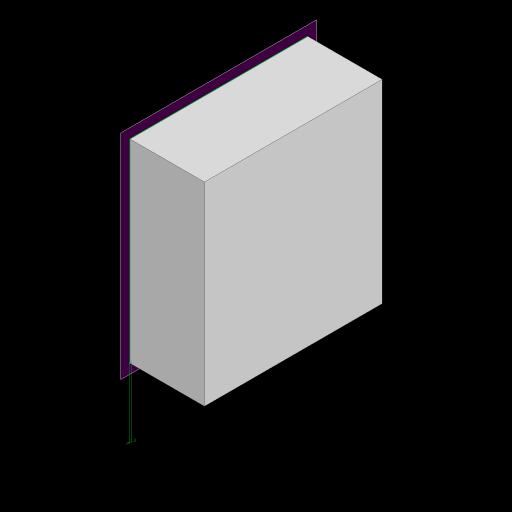
# Autodesk Inventor part: wooferBox
Saved by Autodesk Inventor 2023 (Build 270158000, 158)
## iProperties
Created: 2022-07-12
Part Number: wooferBox
Material: Generic
Document SubType Name: Modeling
Designer: Fuzzyfish
Density: 1 g/cm^3
Appearance: Default
Author: Fuzzyfish
Autodesk Inventor part; units mm, degrees
ref_plane "YZ Plane" through (0, 0, 0) normal (1, 0, 0) x (0, 1, 0)
ref_plane "XZ Plane" through (0, 0, 0) normal (0, 1, 0) x (-1, 0, 0)
ref_plane "XY Plane" through (0, 0, 0) normal (0, 0, 1) x (1, 0, 0)
sketch "Sketch1" plane through (0, 0, 0) normal (0, 1, 0) x (-1, 0, 0)
  line L0 (0, 0) -> (100, 0)
  line L1 (100, 0) -> (100, -119)
  line L2 (100, -119) -> (0, -119)
  line L3 (0, -119) -> (0, 0)
  dimension "d0" = 119
  dimension "d1" = 100
  constraints: 8 end point, 2 parallel, 1 horizontal, 1 perpendicular
  measures "d0" distance between parallel lines of L2 L0
  measures "d1" distance of L1.end L2.end
extrude "Extrusion1" add sketch "Sketch1" along normal blind 130
sketch "Sketch2" plane through (0, 0, -119) normal (0, 0, -1) x (-1, 0, 0)
  circle A0 centre (50, 65) radius 45
  line L0 (100, 0) -> (100, 130) projected
  line L1 (0, 0) -> (0, 130) projected
  line L2 (0, 0) -> (100, 0) projected
  line L3 (0, 130) -> (100, 130) projected
  circle A1 centre (50, 65) radius 36.5
  circle A2 centre (28.0236, 99.1226) radius 1.9
  line L4 (25.6342, 102.8326) -> (74.3658, 27.1674) construction
  line L5 (12.1674, 40.6342) -> (87.8326, 89.3658) construction
  dimension "d6" = 90
  dimension "d7" = 100
  dimension "d8" = 50
  dimension "d9" = 65
  dimension "d10" = 130
  dimension "d11" = 73
  dimension "d12" = 3.8
  constraints: 4 end point, 4 point on circle, 3 centre point, 2 line through centre, 1 coincident, 1 perpendicular, 1 point on line
  measures "d6" diameter of A0
  measures "d7" distance between parallel lines of L0 L1
  measures "d8" distance from line of L1 A0.centre
  measures "d9" distance from line of L2 A0.centre
  measures "d10" distance between parallel lines of L2 L3
  measures "d11" diameter of A1
  measures "d12" diameter of A2
extrude "Extrusion2" cut sketch "Sketch2" against normal blind 8 contours A0 | A1 | A2
extrude "Extrusion3" cut sketch "Sketch2" against normal blind 18 contours A1
ref_plane "Work Plane1" through (-95, 0, -119) normal (-1, 0, 0) x (0, 0, 1)
sketch "Sketch3" plane through (-95, 0, -119) normal (-1, 0, 0) x (0, 0, 1)
  line L0 (18, 28.5) -> (18, 101.5) projected
  line L1 (119, 130) -> (119, 0) projected
  line L2 (119, 0) -> (0, 0) projected
  line L3 (0, 0) -> (0, 65) projected
  line L4 (8, 65) -> (0, 65) projected
  line L5 (0, 130) -> (119, 130) projected
  line L6 (0, 65) -> (0, 130) projected
  line L7 (114, 125) -> (18, 125)
  line L8 (18, 125) -> (18, 5)
  line L9 (18, 5) -> (114, 5)
  line L10 (114, 5) -> (114, 125)
  dimension "d16" = 5
  dimension "d17" = 5
  dimension "d18" = 5
  constraints: 8 end point, 2 parallel, 1 collinear, 1 horizontal, 1 perpendicular
  measures "d16" distance between parallel lines of L2 L9
  measures "d17" distance between parallel lines of L1 L10
  measures "d18" distance between parallel lines of L5 L7
extrude "Extrusion4" cut sketch "Sketch3" against normal blind 90 contours L0 L8 L7 L10 L9
fillet "Fillet1" radius 5 12 edges at (-50, 5, -5) (-5, 5, -53) (-5, 65, -5) (-5, 125, -53) (-50, 125, -5) (-95, 125, -53) (-95, 65, -5) (-95, 5, -53) (-50, 5, -101) (-50, 125, -101) (-95, 65, -101) (-5, 65, -101)
sketch "Sketch8" plane through (-100, 0, -119) normal (-1, 0, 0) x (0, 0, 1)
  point P0 (119, 0)
sketch "Sketch10" plane through (-100, 0, -119) normal (-1, 0, 0) x (0, 0, 1)
  line L0 (0, 0) -> (119, 0) projected
  line L1 (119, 0) -> (119, 130) projected
  line L2 (0, 130) -> (119, 130) projected
  line L3 (0, 0) -> (0, 130) projected
extrude "Extrusion10" add sketch "Sketch10" along normal blind 5
sketch "Sketch12" plane through (0, 130, 0) normal (0, 1, 0) x (1, 0, 0)
  line L0 (0, 119) -> (-105, 119) projected
  line L1 (-105, 0) -> (-105, 119) projected
  line L2 (0, 0) -> (-105, 0) projected
  line L3 (0, 0) -> (0, 119) projected
  line L4 (-105, 0) -> (-100, 0)
  line L5 (-100, 0) -> (-100, 119)
  line L6 (-100, 119) -> (-105, 119)
  line L7 (-105, 119) -> (-105, 0)
  line L8 (-100, 20) -> (-105, 25)
  line L9 (-105, 40) -> (-100, 45)
  line L10 (-105, 94) -> (-100, 99)
  line L11 (-100, 74) -> (-105, 79)
  dimension "d82" = 119
  dimension "d86" = 5
  dimension "d87" = 45
  dimension "d88" = 45
  dimension "d90" = 45
  dimension "d91" = 45
  dimension "d92" = 20
  dimension "d93" = 25
  dimension "d94" = 20
  dimension "d95" = 25
  constraints: 16 end point, 9 point on line, 2 parallel, 1 horizontal, 1 perpendicular
  measures "d82" distance of L0.end L1.start
  measures "d86" distance between parallel lines of L1 L5
  measures "d87" angle of L5 L8
  measures "d88" angle of L5 L9
  measures "d90" angle of L5 L11
  measures "d91" angle of L5 L10
  measures "d92" distance of L4.end L8.start
  measures "d93" distance of L9.end L8.start
  measures "d94" distance of L5.end L10.end
  measures "d95" distance of L11.start L10.end
extrude "Extrusion11" cut sketch "Sketch12" against normal blind 127 contours L5 L11 L1 L10 | L8 L1 L9 L5
fillet "Fillet2" radius 1 8 edges at (-105, 66.5, -25) (-100, 66.5, -20) (-105, 66.5, -40) (-100, 66.5, -45) (-105, 66.5, -79) (-100, 66.5, -74) (-105, 66.5, -94) (-100, 66.5, -99)
sketch "Sketch13" plane through (-10, 120, -5) normal (0, 0, -1) x (-1, 0, 0)
  line L0 (82.5, 0) -> (-2.5, 0)
  line L1 (-2.5, 0) -> (-2.5, -110)
  line L2 (-2.5, -110) -> (82.5, -110)
  line L3 (82.5, -110) -> (82.5, 0)
  line L4 (-5, 0) -> (-5, -110) projected
  line L5 (85, -110) -> (85, 0) projected
  circle A0 centre (78.5, -4.3) radius 1.8
  circle A1 centre (78.5, -4.3) radius 2.5
  line L6 (78.5, -4.3) -> (78.5, -140.0823) construction
  line L7 (78.5, -4.3) -> (-34.9987, -4.3) construction
  line L8 (1.5, 27.6777) -> (1.5, -220.2724) construction
  line L9 (-45.8754, -105.7) -> (99.6232, -105.7) construction
  line L10 (80, 5) -> (0, 5) construction
  line L11 (0, -115) -> (80, -115) construction
  circle A2 centre (78.5, -105.7) radius 1.8
  circle A3 centre (78.5, -105.7) radius 2.5
  circle A4 centre (1.5, -105.7) radius 1.8
  circle A5 centre (1.5, -105.7) radius 2.5
  circle A6 centre (1.5, -4.3) radius 1.8
  circle A7 centre (1.5, -4.3) radius 2.5
  point P0 (-10, -120)
  dimension "d97" = 85
  dimension "d98" = 110
  dimension "d99" = 90
  dimension "d100" = 2.5
  dimension "d101" = 4
  dimension "d102" = 4.3
  dimension "d103" = 3.6
  dimension "d104" = 5
  dimension "d105" = 4.3
  dimension "d107" = 120
  dimension "d108" = 5
  dimension "d109" = 4
  dimension "d110" = 3.6
  dimension "d111" = 5
  dimension "d112" = 3.6
  dimension "d113" = 5
  dimension "d114" = 3.6
  dimension "d115" = 5
  constraints: 16 end point, 8 centre point, 7 coincident, 6 point on line, 3 horizontal, 2 parallel, 2 vertical, 1 perpendicular
  measures "d97" distance of L1.end L2.end
  measures "d98" distance of L0.end L1.end
  measures "d99" distance between parallel lines of L4 L5
  measures "d100" distance between parallel lines of L5 L3
  measures "d101" distance from line of L3 A0.centre
  measures "d102" distance from line of L0 A0.centre
  measures "d103" diameter of A0
  measures "d104" diameter of A1
  measures "d105" distance between parallel lines of L2 L9
  measures "d107" distance between parallel lines of L10 L11
  measures "d108" distance between parallel lines of L11 L2
  measures "d109" distance between parallel lines of L8 L1
  measures "d110" diameter of A2
  measures "d111" diameter of A3
  measures "d112" diameter of A4
  measures "d113" diameter of A5
  measures "d114" diameter of A6
  measures "d115" diameter of A7
extrude "Extrusion12" add sketch "Sketch13" along normal blind 3 contours A1 | A3 | A5 | A7
sketch "Sketch14" plane through (-105, 0, -119) normal (-1, 0, 0) x (0, 0, 1)
  line L0 (19.5, 52) -> (19.5, 34) construction
  line L1 (18, 52) -> (18, 34)
  line L2 (21, 34) -> (21, 52)
  arc A0 (21, 52) -> (18, 52) centre (19.5, 52) ccw
  arc A1 (18, 34) -> (21, 34) centre (19.5, 34) ccw
  line L3 (0, 130) -> (0, 0) projected
  line L4 (0, 0) -> (119, 0) projected
  point P0 (19.5, 43)
  dimension "d118" = 18
  dimension "d119" = 3
  dimension "d121" = 18
  dimension "d122" = 34
  constraints: 8 end point, 4 point on circle, 4 tangent, 2 centre point, 1 midpoint, 1 parallel, 1 vertical
  measures "d118" distance of L0.start L0.end
  measures "d119" distance between parallel lines of L1 L2
  measures "d121" distance between parallel lines of L3 L1
  measures "d122" distance from line of L4 L0.end
extrude "Extrusion13" cut sketch "Sketch14" against normal blind 20
sketch "Sketch15" plane through (-50, 65, -111) normal (0, 0, -1) x (-1, 0, 0)
  circle A0 centre (0, 0) radius 45 construction
  line L0 (31.8198, 31.8198) -> (-31.8198, -31.8198) construction
  line L1 (31.8198, -31.8198) -> (-31.8198, 31.8198) construction
  circle A1 centre (0, 0) radius 36.5 construction
  circle A2 centre (0, 0) radius 40.75 construction
  line L2 (0, -45) -> (0, 45) construction
  line L3 (-40, -60) -> (40, -60) construction
  circle A3 centre (28.8146, 28.8146) radius 1.8
  circle A4 centre (-28.8146, 28.8146) radius 1.8
  circle A5 centre (28.8146, -28.8146) radius 1.8
  circle A6 centre (-28.8146, -28.8146) radius 1.8
  point P0 (-50, -65)
  dimension "d125" = 45
  dimension "d126" = 73
  dimension "d129" = 90
  dimension "d130" = 4.25
  dimension "d131" = 3.6
  dimension "d135" = 3.6
  dimension "d136" = 3.6
  dimension "d137" = 3.6
  constraints: 10 point on circle, 6 end point, 5 centre point, 5 coincident, 4 point on line, 2 midpoint, 2 perpendicular
  measures "d125" angle of L0 L2
  measures "d126" diameter of A1
  measures "d129" diameter of A0
  measures "d130" radial gap between concentric circles of A1 A2
  measures "d131" diameter of A3
  measures "d135" diameter of A4
  measures "d136" diameter of A5
  measures "d137" diameter of A6
extrude "Extrusion14" cut sketch "Sketch15" against normal blind 40
ref_plane "Work Plane2" through (-50, 0, -119) normal (-1, 0, 0) x (0, 0, 1)
split "Split1" plane through (-50, 0, -119) removes the side toward (-1, 0, 0)
sketch "Sketch18" plane through (-50, 0, -119) normal (-1, 0, 0) x (0, 0, 1)
  line L0 (8, 110) -> (0, 110) projected
  line L1 (8, 101.5) -> (8, 110) projected
  line L2 (18, 101.5) -> (8, 101.5) projected
  line L3 (18, 120) -> (18, 101.5) projected
  arc A0 (23, 125) -> (18, 120) centre (23, 120) ccw projected
  line L4 (109, 125) -> (23, 125) projected
  arc A1 (114, 120) -> (109, 125) centre (109, 120) ccw projected
  line L5 (114, 10) -> (114, 120) projected
  arc A2 (109, 5) -> (114, 10) centre (109, 10) ccw projected
  line L6 (23, 5) -> (109, 5) projected
  arc A3 (18, 10) -> (23, 5) centre (23, 10) ccw projected
  line L7 (18, 28.5) -> (18, 10) projected
  line L8 (8, 28.5) -> (18, 28.5) projected
  line L9 (8, 20) -> (8, 28.5) projected
  line L10 (0, 20) -> (8, 20) projected
  line L11 (0, 0) -> (0, 20) projected
  line L12 (119, 0) -> (0, 0) projected
  line L13 (119, 130) -> (119, 0) projected
  line L14 (0, 130) -> (119, 130) projected
  line L15 (0, 110) -> (0, 130) projected
  line L16 (117.7, 1.3) -> (1.3, 1.3)
  line L17 (1.3, 1.3) -> (1.3, 18.7)
  line L18 (1.3, 18.7) -> (9.3, 18.7)
  line L19 (9.3, 18.7) -> (9.3, 27.2)
  line L20 (9.3, 27.2) -> (16.7, 27.2)
  line L21 (16.7, 27.2) -> (16.7, 10)
  arc A4 (16.7, 10) -> (23, 3.7) centre (23, 10) ccw
  line L22 (23, 3.7) -> (109, 3.7)
  arc A5 (109, 3.7) -> (115.3, 10) centre (109, 10) ccw
  line L23 (115.3, 10) -> (115.3, 120)
  arc A6 (115.3, 120) -> (109, 126.3) centre (109, 120) ccw
  line L24 (109, 126.3) -> (23, 126.3)
  arc A7 (23, 126.3) -> (16.7, 120) centre (23, 120) ccw
  line L25 (16.7, 120) -> (16.7, 102.8)
  line L26 (16.7, 102.8) -> (9.3, 102.8)
  line L27 (9.3, 102.8) -> (9.3, 111.3)
  line L28 (9.3, 111.3) -> (1.3, 111.3)
  line L29 (1.3, 111.3) -> (1.3, 128.7)
  line L30 (1.3, 128.7) -> (117.7, 128.7)
  line L31 (117.7, 128.7) -> (117.7, 1.3)
  dimension "d140" = 1.3
  constraints: 32 end point, 8 point on circle, 4 centre point, 19 other
  measures "d140" distance between parallel lines of L13 L31
equation "\"d8\" = 0.5 * d7"
equation "\"d9\" = 0.5 * d10"
equation "\"d100\" = -0.5 * d97 + 0.5 * d99"
equation "\"d108\" = -0.5 * d98 + 0.5 * d107"
equation "\"d130\" = -0.25 * d126 + 0.25 * d129"
equation "\"d135\" = d131"
equation "\"d136\" = d131"
equation "\"d137\" = d131"
body "Solid1"
